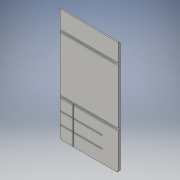
# Autodesk Inventor part: Left Side
Saved by Autodesk Inventor 2016 (Build 200138000, 138)
## iProperties
Created: 2017-10-30
Part Number: Left Side
Material: Generic
Document SubType Name: Modeling
Designer: mathaetaes
Density: 1 g/cm^3
Appearance: Default
Author: mathaetaes
Autodesk Inventor part; units mm, degrees
ref_plane "YZ Plane" through (0, 0, 0) normal (1, 0, 0) x (0, 1, 0)
ref_plane "XZ Plane" through (0, 0, 0) normal (0, 1, 0) x (-1, 0, 0)
ref_plane "XY Plane" through (0, 0, 0) normal (0, 0, 1) x (1, 0, 0)
sketch "Sketch1" plane through (0, 0, 0) normal (0, 0, 1) x (1, 0, 0)
  line L0 (-222.9556, 663.6813) -> (246.9444, 663.6813)
  line L1 (246.9444, 663.6813) -> (246.9444, -238.0187)
  line L2 (246.9444, -238.0187) -> (-222.9556, -238.0187)
  line L3 (-222.9556, -238.0187) -> (-222.9556, 663.6813)
  point P0 (0, 0)
  dimension "d0" = 469.9
  dimension "d1" = 901.7
  constraints: 8 end point, 2 parallel, 1 horizontal, 1 perpendicular
  measures "d0" distance of L1.end L2.end
  measures "d1" distance of L0.end L1.end
extrude "Board" add sketch "Sketch1" along normal blind 19.05
sketch "Sketch6" plane through (0, 0, 0) normal (0, 0, -1) x (-1, 0, 0)
  line L0 (222.9556, 663.6813) -> (-246.9444, 663.6813) projected
  line L1 (-246.9444, 663.6813) -> (222.9556, 663.6813)
  line L2 (222.9556, 663.6813) -> (222.9556, 650.9813)
  line L3 (222.9556, 650.9813) -> (-246.9444, 650.9813)
  line L4 (-246.9444, 650.9813) -> (-246.9444, 663.6813)
  line L5 (-246.9444, -238.0187) -> (222.9556, -238.0187)
  line L6 (222.9556, -238.0187) -> (222.9556, -228.4937)
  line L7 (222.9556, -228.4937) -> (-246.9444, -228.4937)
  line L8 (-246.9444, -228.4937) -> (-246.9444, -238.0187)
  line L9 (-246.9444, -238.0187) -> (222.9556, -238.0187) projected
  line L10 (222.9556, -238.0187) -> (222.9556, 663.6813) projected
  point P0 (0, 0)
  dimension "d28" = 12.7
  dimension "d37" = 9.525
  constraints: 16 end point, 4 parallel, 3 collinear, 2 horizontal, 2 perpendicular, 1 point on line
  measures "d28" distance of L1.end L2.end
  measures "d37" distance between parallel lines of L5 L7
extrude "Top and Bottom Exterior Dados" cut sketch "Sketch6" against normal blind 9.525
sketch "Sketch2" plane through (0, 0, 19.05) normal (0, 0, 1) x (1, 0, 0)
  line L0 (-222.9556, 663.6813) -> (-222.9556, -238.0187) projected
  line L1 (246.9444, -238.0187) -> (246.9444, 663.6813) projected
  line L2 (-222.9556, 69.9563) -> (246.9444, 69.9563)
  line L3 (246.9444, 69.9563) -> (246.9444, 50.9063)
  line L4 (246.9444, 50.9063) -> (-222.9556, 50.9063)
  line L5 (-222.9556, 50.9063) -> (-222.9556, 69.9563)
  line L6 (246.9444, 663.6813) -> (-222.9556, 663.6813) projected
  line L7 (-222.9556, -238.0187) -> (246.9444, -238.0187) projected
  point P0 (0, 0)
  dimension "d4" = 19.05
  dimension "d16" = 288.925
  constraints: 8 end point, 2 parallel, 2 point on line, 1 horizontal, 1 perpendicular
  measures "d4" distance between parallel lines of L4 L2
  measures "d16" distance between parallel lines of L7 L4
extrude "Lower Inner Dado" cut sketch "Sketch2" against normal blind 9.525 contours L2 L1 L4 L0
sketch "Sketch4" plane through (0, 0, 19.05) normal (0, 0, 1) x (1, 0, 0)
  line L0 (-222.9556, 523.9813) -> (246.9444, 523.9813)
  line L1 (246.9444, 523.9813) -> (246.9444, 504.9313)
  line L2 (246.9444, 504.9313) -> (-222.9556, 504.9313)
  line L3 (-222.9556, 504.9313) -> (-222.9556, 523.9813)
  line L4 (-222.9556, 663.6813) -> (246.9444, 663.6813) projected
  line L5 (-222.9556, 663.6813) -> (-222.9556, 69.9563) projected
  line L6 (246.9444, 69.9563) -> (246.9444, 663.6813) projected
  line L7 (-222.9556, 650.9813) -> (246.9444, 650.9813) projected
  point P0 (0, 0)
  dimension "d18" = 19.05
  dimension "d36" = 127
  constraints: 8 end point, 2 collinear, 2 parallel, 1 horizontal, 1 perpendicular
  measures "d18" distance of L0.end L1.end
  measures "d36" distance between parallel lines of L7 L0
extrude "Top Inner Dado" cut sketch "Sketch4" against normal blind 9.525 contours L0 L1 L2 L3
sketch "Sketch3" plane through (0, 0, 19.05) normal (0, 0, 1) x (1, 0, 0)
  line L0 (-222.9556, -133.2437) -> (119.9444, -133.2437)
  line L1 (119.9444, -133.2437) -> (119.9444, -139.5937)
  line L2 (119.9444, -139.5937) -> (-222.9556, -139.5937)
  line L3 (-222.9556, -139.5937) -> (-222.9556, -133.2437)
  line L4 (-222.9556, -238.0187) -> (246.9444, -238.0187) projected
  line L5 (-222.9556, -37.9937) -> (119.9444, -37.9937)
  line L6 (119.9444, -37.9937) -> (119.9444, -44.3437)
  line L7 (119.9444, -44.3437) -> (-222.9556, -44.3437)
  line L8 (-222.9556, -44.3437) -> (-222.9556, -37.9937)
  line L9 (-222.9556, 50.9063) -> (-222.9556, -238.0187) projected
  line L10 (246.9444, -238.0187) -> (246.9444, 50.9063) projected
  line L11 (246.9444, -228.4937) -> (-222.9556, -228.4937) projected
  line L12 (246.9444, 50.9063) -> (-222.9556, 50.9063) projected
  point P0 (0, 0)
  dimension "d9" = 6.35
  dimension "d12" = 6.35
  dimension "d13" = 88.9
  dimension "d21" = 127
  dimension "d23" = 127
  dimension "d65" = 88.9
  constraints: 16 end point, 4 parallel, 2 collinear, 2 horizontal, 2 perpendicular
  measures "d9" distance of L0.end L1.end
  measures "d12" distance of L5.end L6.end
  measures "d13" distance between parallel lines of L0 L7
  measures "d21" distance between parallel lines of L6 L10
  measures "d23" distance between parallel lines of L10 L1
  measures "d65" distance between parallel lines of L11 L2
extrude "Wine Bottle Dados" cut sketch "Sketch3" against normal blind 6.35 contours L0 L1 L2 L3 | L8 L5 L6 L7
sketch "Sketch7" plane through (0, 0, 19.05) normal (0, 0, 1) x (1, 0, 0)
  line L0 (246.9444, 50.9063) -> (-222.9556, 50.9063) projected
  line L1 (-108.6556, -238.0187) -> (-115.0056, -238.0187)
  line L2 (-115.0056, -238.0187) -> (-115.0056, 50.9063)
  line L3 (-115.0056, 50.9063) -> (-108.6556, 50.9063)
  line L4 (-108.6556, 50.9063) -> (-108.6556, -238.0187)
  line L5 (119.9444, -37.9937) -> (119.9444, -44.3437) projected
  line L6 (-222.9556, -238.0187) -> (246.9444, -238.0187) projected
  point P0 (0, 0)
  dimension "d31" = 6.35
  dimension "d32" = 228.6
  constraints: 8 end point, 2 parallel, 1 collinear, 1 horizontal, 1 perpendicular, 1 point on line
  measures "d31" distance of L1.start L1.end
  measures "d32" distance between parallel lines of L4 L5
extrude "Wine Rack Back Vertical Dado" cut sketch "Sketch7" against normal blind 9.525
sketch "Sketch8" plane through (-222.9556, -228.4937, 0) normal (-1, 0, 0) x (0, 0, 1)
  line L0 (19.05, 892.175) -> (9.525, 892.175)
  line L1 (9.525, 892.175) -> (9.525, -9.525)
  line L2 (9.525, -9.525) -> (19.05, -9.525)
  line L3 (19.05, -9.525) -> (19.05, 892.175)
  line L4 (9.525, 892.175) -> (19.05, 892.175) projected
  line L5 (9.525, -9.525) -> (19.05, -9.525) projected
  line L6 (19.05, 733.425) -> (19.05, 298.45) projected
  point P0 (0, 228.4937)
  point P1 (19.05, 184.15)
  point P2 (19.05, 95.25)
  dimension "d39" = 9.525
  constraints: 8 end point, 3 collinear, 2 parallel, 1 horizontal, 1 perpendicular
  measures "d39" distance of L1.end L2.end
extrude "Vertical Backing Dado" cut sketch "Sketch8" against normal blind 6.35
sketch "Sketch9" plane through (0, 0, 0) normal (0, 0, -1) x (-1, 0, 0)
  line L0 (83.2556, 650.9813) -> (121.3556, 650.9813)
  line L1 (121.3556, 650.9813) -> (121.3556, 630.3438)
  line L2 (118.1806, 627.1688) -> (86.4306, 627.1688)
  line L3 (83.2556, 630.3438) -> (83.2556, 650.9813)
  line L4 (222.9556, 650.9813) -> (-246.9444, 650.9813) projected
  line L5 (222.9556, -228.4937) -> (222.9556, 650.9813) projected
  line L6 (-158.0444, 650.9813) -> (-119.9444, 650.9813)
  line L7 (-119.9444, 650.9813) -> (-119.9444, 630.3438)
  line L8 (-123.1194, 627.1688) -> (-154.8694, 627.1688)
  line L9 (-158.0444, 630.3438) -> (-158.0444, 650.9813)
  arc A0 (-158.0444, 630.3438) -> (-154.8694, 627.1688) centre (-154.8694, 630.3438) ccw
  arc A1 (-123.1194, 627.1688) -> (-119.9444, 630.3438) centre (-123.1194, 630.3438) ccw
  arc A2 (83.2556, 630.3438) -> (86.4306, 627.1688) centre (86.4306, 630.3438) ccw
  arc A3 (118.1806, 627.1688) -> (121.3556, 630.3438) centre (118.1806, 630.3438) ccw
  point P0 (0, 0)
  point P1 (121.3556, 627.1688)
  point P2 (83.2556, 627.1688)
  point P3 (-119.9444, 627.1688)
  point P4 (-158.0444, 627.1688)
  dimension "d42" = 38.1
  dimension "d43" = 23.8125
  dimension "d44" = 101.6
  dimension "d45" = 38.1
  dimension "d46" = 23.8125
  dimension "d47" = 203.2
  dimension "d48" = 3.175
  constraints: 16 end point, 8 point on circle, 8 point on line, 8 tangent, 4 centre point, 4 parallel, 3 equal radius, 2 collinear, 2 horizontal, 2 perpendicular
  measures "d42" distance of point (121.356, 627.169) point (83.256, 627.169)
  measures "d43" distance of L0.end point (121.356, 627.169)
  measures "d44" distance between parallel lines of L5 L1
  measures "d45" distance of point (-119.944, 627.169) point (-158.044, 627.169)
  measures "d46" distance of L6.end point (-119.944, 627.169)
  measures "d47" distance between parallel lines of L3 L7
  measures "d48" radius of A0
extrude "Top Hinge Notch" cut sketch "Sketch9" against normal blind 3.175
sketch "Sketch11" plane through (246.9444, -238.0187, 19.05) normal (1, 0, 0) x (0, 0, -1)
  line L0 (9.525, 9.525) -> (19.05, 9.525) projected
  line L1 (0, 0) -> (9.525, 0)
  line L2 (9.525, 0) -> (9.525, 9.525)
  line L3 (9.525, 9.525) -> (0, 9.525)
  line L4 (0, 9.525) -> (0, 0)
  point P0 (19.05, 238.0187)
  constraints: 8 end point, 2 parallel, 1 horizontal, 1 perpendicular
extrude "Front notch to cover dado" cut sketch "Sketch11" against normal blind 6.35
sketch "Sketch12" plane through (0, 0, 9.525) normal (0, 0, -1) x (-1, 0, 0)
  line L0 (216.6056, -228.4937) -> (222.9556, -228.4937) projected
  line L1 (216.6056, -238.0187) -> (-240.5944, -238.0187) projected
  line L2 (222.9556, -228.4937) -> (203.9056, -228.4937)
  line L3 (203.9056, -228.4937) -> (203.9056, -238.0187)
  line L4 (203.9056, -238.0187) -> (222.9556, -238.0187)
  line L5 (222.9556, -238.0187) -> (222.9556, -228.4937)
  point P0 (0, 0)
  point P1 (115.0056, -238.0187)
  dimension "d62" = 19.05
  constraints: 8 end point, 2 parallel, 1 horizontal, 1 perpendicular, 1 point on line
  measures "d62" distance of L3.end L4.end
extrude "Rear notch for runner" cut sketch "Sketch12" against normal blind 19.05
equation "\"d6\" = 0.5 * d2"
equation "\"d33\" = 0.5 * d2"
equation "\"d39\" = 0.5 * d2"
equation "\"d45\" = d42"
equation "\"d46\" = d43"
equation "\"d47\" = 2 * d44"
equation "\"d2\" = 19.05"
body "Solid1"
